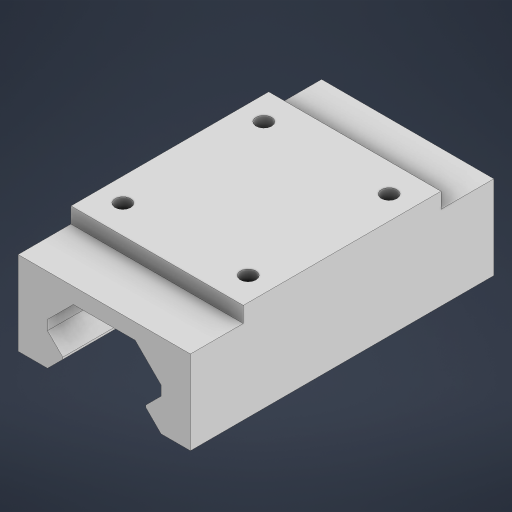
# Autodesk Inventor part: HGH20CA Slider Block
Saved by Autodesk Inventor 2024.2 (Build 282272000, 272)
## iProperties
Created: 2024-10-04
Part Number: HGH20CA Slider Block
Material: Generic
Document SubType Name: Modeling
Designer: jerem
Density: 1 g/cm^3
Appearance: Default
Author: jerem
Autodesk Inventor part; units mm, degrees
ref_plane "YZ Plane" through (0, 0, 0) normal (1, 0, 0) x (0, 1, 0)
ref_plane "XZ Plane" through (0, 0, 0) normal (0, 1, 0) x (-1, 0, 0)
ref_plane "XY Plane" through (0, 0, 0) normal (0, 0, 1) x (1, 0, 0)
sketch "Sketch1" plane through (0, 0, 0) normal (0, 0, 1) x (1, 0, 0)
  line L0 (0, 0) -> (-22, 0)
  line L1 (-22, 0) -> (-22, 0)
  line L2 (-22, 0) -> (-14.5, 0)
  line L3 (-22, 0) -> (-22, 25.4)
  line L4 (-22, 25.4) -> (0, 25.4)
  line L5 (-29.0722, -4.6) -> (-18.7593, -4.6) construction
  line L6 (-22, 0) -> (0, 0) construction
  line L7 (0, 0) -> (22, 0) construction
  line L8 (0, -10.6) -> (0, 31.4) construction
  line L9 (0, -4.6) -> (0, 12.9) construction
  line L10 (0, -4.6) -> (-10, -4.6) construction
  line L11 (0, -4.6) -> (10, -4.6) construction
  line L12 (-10, -4.6) -> (-10, 0) construction
  line L13 (-10, 0) -> (-6.1, 3.9) construction
  line L14 (-6.1, 3.9) -> (-6.1, 4.4) construction
  line L15 (-6.1, 4.4) -> (-10, 8.3) construction
  line L16 (-10, 8.3) -> (-10, 10.8) construction
  line L17 (-10, 10.8) -> (-7.9, 12.9) construction
  line L18 (-7.9, 12.9) -> (0, 12.9) construction
  line L19 (10, 0) -> (6.1, 3.9) construction
  line L20 (6.1, 3.9) -> (6.1, 4.4) construction
  line L21 (6.1, 4.4) -> (10, 8.3) construction
  line L22 (10, 8.3) -> (10, 10.8) construction
  line L23 (10, 10.8) -> (7.9, 12.9) construction
  line L24 (10, -4.6) -> (10, 0) construction
  line L25 (7.9, 12.9) -> (0, 12.9) construction
  line L26 (-14.5, 8.3) -> (-14.5, 10.8)
  line L27 (-14.5, 10.8) -> (-7.9, 17.4)
  line L28 (-7.9, 17.4) -> (0, 17.4)
  line L29 (-14.5, 0) -> (-10.6, 3.9)
  line L30 (-10.6, 3.9) -> (-10.6, 4.4)
  line L31 (-10.6, 4.4) -> (-14.5, 8.3)
  line L32 (-10.6, 3.9) -> (-6.1, 3.9) construction
  line L33 (-10, 8.3) -> (-14.5, 8.3) construction
  line L34 (22, 0) -> (14.5, 0)
  line L35 (22, 0) -> (22, 25.4)
  line L36 (22, 25.4) -> (0, 25.4)
  line L37 (14.5, 8.3) -> (14.5, 10.8)
  line L38 (14.5, 10.8) -> (7.9, 17.4)
  line L39 (7.9, 17.4) -> (0, 17.4)
  line L40 (14.5, 0) -> (10.6, 3.9)
  line L41 (10.6, 3.9) -> (10.6, 4.4)
  line L42 (10.6, 4.4) -> (14.5, 8.3)
  point P0 (-3.95, 17.4)
  dimension "d0" = 4.6
  dimension "d1" = 44
  dimension "d3" = 17.5
  dimension "d4" = 20
  dimension "d5" = 4.6
  dimension "d6" = 8.5
  dimension "d7" = 135
  dimension "d8" = 0.5
  dimension "d9" = 135
  dimension "d10" = 2.5
  dimension "d11" = 7.5
  dimension "d12" = 25.4
  dimension "d13" = 45
  dimension "d14" = 135
  dimension "d15" = 2.5
  dimension "d16" = 0.5
  dimension "d17" = 135
  dimension "d19" = 4.5
  constraints: 84 end point, 14 symmetric about line, 9 horizontal, 8 point on line, 5 vertical, 4 perpendicular, 3 collinear, 2 parallel, 1 midpoint
  measures "d0" distance from line of L0.end L5
  measures "d1" distance of L7.end L0.end
  measures "d3" distance of L11.start L25.end
  measures "d4" distance of L11.end L10.end
  measures "d5" distance of L10.end L13.start
  measures "d6" distance from line of L15.start L18
  measures "d7" angle of L18 L17
  measures "d8" distance of L13.end L15.start
  measures "d9" angle of L14 L15
  measures "d10" distance of L16.start L17.start
  measures "d11" distance of L1.end L2.end
  measures "d12" distance of L1.end L3.end
  measures "d13" angle of L0 L29
  measures "d14" angle of L31 L26
  measures "d15" distance of L26.start L26.end
  measures "d16" distance of L29.end L30.end
  measures "d17" angle of L26 L27
  measures "d19" distance between parallel lines of L18 L28
extrude "Extrusion1" add sketch "Sketch1" along normal blind 77.5
sketch "Sketch2" plane through (-22, 25.4, 0) normal (0, 1, 0) x (1, 0, 0)
  circle A0 centre (6, -20.75) radius 2
  circle A1 centre (6, -56.75) radius 2
  line L0 (6, -20.75) -> (6, -56.75)
  circle A2 centre (38, -20.75) radius 2
  circle A3 centre (38, -56.75) radius 2
  line L1 (38, -20.75) -> (38, -56.75) construction
  line L2 (22, 0) -> (22, -77.5) construction
  line L3 (44, -77.5) -> (0, -77.5) construction
  line L4 (38, -38.75) -> (22, -38.75) construction
  line L5 (6, -38.75) -> (22, -38.75) construction
  line L6 (0, 0) -> (0, -77.5) construction
  line L7 (44, -64) -> (0, -64) construction
  line L8 (0, -64) -> (0, -13.5) construction
  line L9 (0, -13.5) -> (44, -13.5) construction
  line L10 (44, -13.5) -> (44, -64) construction
  line L11 (44, -64) -> (0, -13.5) construction
  line L12 (0, -64) -> (44, -13.5) construction
  line L13 (44, 0) -> (44, -77.5) projected
  line L14 (0, -13.5) -> (44, -13.5)
  line L15 (44, -13.5) -> (44, 0)
  line L16 (44, 0) -> (0, 0)
  line L17 (0, 0) -> (0, -13.5)
  line L18 (0, -64) -> (44, -64)
  line L19 (44, -64) -> (44, -77.5)
  line L20 (44, -77.5) -> (0, -77.5)
  line L21 (0, -77.5) -> (0, -64)
  point P0 (7.5, -77.5)
  dimension "d22" = 36
  dimension "d23" = 4
  dimension "d24" = 4
  dimension "d25" = 36
  dimension "d26" = 4
  dimension "d27" = 4
  dimension "d29" = 32
  dimension "d30" = 50.5
  constraints: 38 end point, 7 equal length, 7 midpoint, 5 horizontal, 4 centre point, 4 perpendicular, 1 collinear, 1 point on line
  measures "d22" distance of L0.start L0.end
  measures "d23" diameter of A0
  measures "d24" diameter of A1
  measures "d25" distance of L1.start L1.end
  measures "d26" diameter of A2
  measures "d27" diameter of A3
  measures "d29" distance between parallel lines of L1 L0
  measures "d30" distance between parallel lines of L7 L9
extrude "Extrusion2" cut sketch "Sketch2" against normal blind 8 contours A0 | A1 | A2 | A3
extrude "Extrusion3" cut sketch "Sketch2" against normal blind 4 contours L13 L20 L21 L18 | L13 L14 L17 L16
equation "\"d15\" = d10"
equation "\"d16\" = d8"
body "Solid1"
